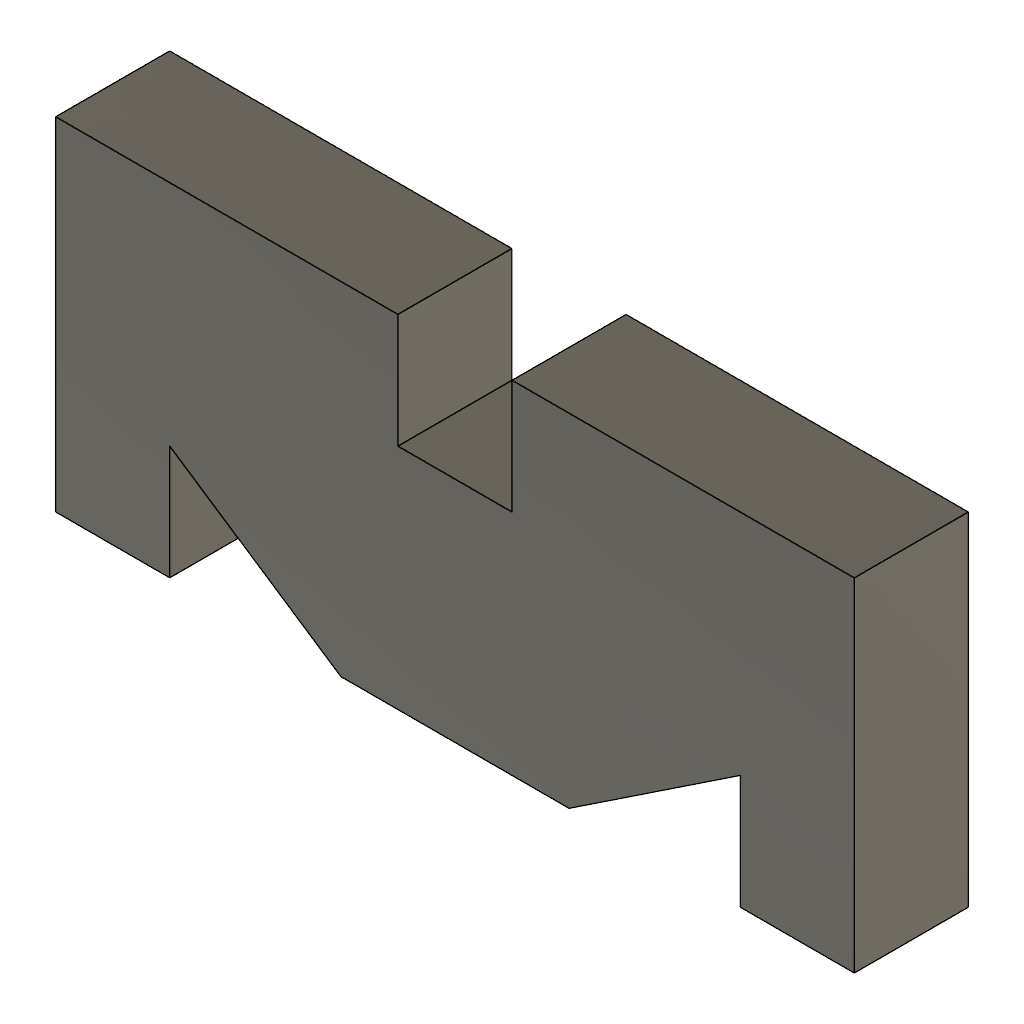
exercise 6 (Autodesk Fusion 360 design; units mm, degrees)
part number: 2026-10-03-23-22-25-951
Autodesk Fusion 360 part; units mm, degrees
sketch "Sketch1" plane through (0, 0, 0) normal (0, 1, 0) x (1, 0, 0)
  line L0 (20, -30) -> (-10, -30)
  line L1 (-10, -30) -> (-10, 0)
  line L2 (0, 0) -> (0, -10)
  line L3 (0, -10) -> (15, 0)
  line L4 (15, 0) -> (25, 0)
  line L5 (20, -30) -> (20, -20)
  line L6 (20, -20) -> (25, -20)
  line L7 (-10, 0) -> (0, 0)
  line L8 (50, 0) -> (50, -10)
  line L9 (60, 0) -> (50, 0)
  line L10 (50, -10) -> (35, 0)
  line L11 (60, -30) -> (60, 0)
  line L12 (30, -30) -> (60, -30)
  line L13 (35, 0) -> (25, 0)
  line L14 (30, -30) -> (30, -20)
  line L15 (30, -20) -> (25, -20)
  point P0 (50, 0)
  dimension "d14" = 30
  dimension "d15" = 30
  dimension "d18" = 10
  dimension "d19" = 15
  dimension "d20" = 10
  dimension "d21" = 15
  dimension "d22" = 10
  dimension "d23" = 5
  dimension "d25" = 10
  constraint coincident L2.start L7.end
  constraint perpendicular L2 L4
  constraint perpendicular L0 L5
  constraint perpendicular L5 L6
  constraint perpendicular L1 L7
  measures "d14" distance of L0.end L1.end
  measures "d15" distance of L0.start L0.end
  measures "d18" distance of L2.start L2.end
  measures "d19" distance of L2.start L3.end
  measures "d20" distance of L3.end L4.end
  measures "d21" horizontal distance of L2.end L3.end
  measures "d22" distance of L0.start L5.end
  measures "d23" distance of L5.end L6.end
  measures "d25" distance of L1.end L2.start
extrude "Extrude1" add sketch "Sketch1" along normal blind 10
